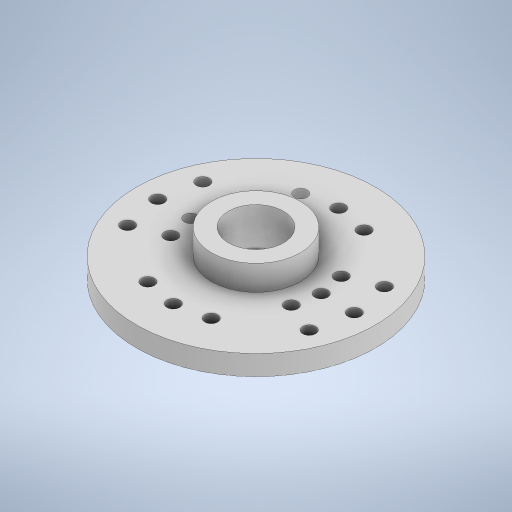
# Autodesk Inventor part: Standard Servo Horn - White Circle
Saved by Autodesk Inventor 2023 (Build 270158000, 158)
## iProperties
Created: 2023-09-05
Part Number: Standard Servo Horn - White Circle
Material: Generic
Document SubType Name: Modeling
Designer: Nate
Density: 1 g/cm^3
Appearance: Default
Author: Nate
Autodesk Inventor part; units mm, degrees
ref_plane "YZ Plane" through (0, 0, 0) normal (1, 0, 0) x (0, 1, 0)
ref_plane "XZ Plane" through (0, 0, 0) normal (0, 1, 0) x (-1, 0, 0)
ref_plane "XY Plane" through (0, 0, 0) normal (0, 0, 1) x (1, 0, 0)
sketch "Sketch1" plane through (0, 0, 0) normal (0, 1, 0) x (-1, 0, 0)
  circle A0 centre (0, 0) radius 11.915
  circle A1 centre (0, 0) radius 9.8
  circle A2 centre (0, 0) radius 8.25
  circle A3 centre (0, 0) radius 6.5
  circle A4 centre (6.5, 0) radius 0.65
  circle A5 centre (9.8, 0) radius 0.65
  circle A6 centre (9.054, 3.7503) radius 0.65
  circle A7 centre (6.0052, 2.4874) radius 0.65
  circle A8 centre (9.054, -3.7503) radius 0.65
  circle A9 centre (6.0052, -2.4874) radius 0.65
  circle A10 centre (-9.054, -3.7503) radius 0.65
  circle A11 centre (-6.0052, -2.4874) radius 0.65
  circle A12 centre (-6.5, 0) radius 0.65
  circle A13 centre (-9.8, 0) radius 0.65
  circle A14 centre (-6.0052, 2.4874) radius 0.65
  circle A15 centre (-9.054, 3.7503) radius 0.65
  circle A16 centre (0, 8.25) radius 0.65
  circle A17 centre (-3.1571, 7.622) radius 0.65
  circle A18 centre (3.1571, 7.622) radius 0.65
  circle A19 centre (-3.1571, -7.622) radius 0.65
  circle A20 centre (0, -8.25) radius 0.65
  circle A21 centre (3.1571, -7.622) radius 0.65
  circle A22 centre (0, 0) radius 1.37
  circle A23 centre (0, 0) radius 2.75
  circle A24 centre (0, 0) radius 2.97
  circle A25 centre (0, 0) radius 3.73
  circle A26 centre (0, 0) radius 4.44
  dimension "d1" = 19.6
  dimension "d2" = 16.5
  dimension "d3" = 13
  dimension "d0" = 23.83
  dimension "d4" = 1.3
  dimension "d5" = 1.3
  dimension "d8" = 22.5
  dimension "d12" = 337.5
  dimension "d16" = 180
  dimension "d18" = 1.3
  dimension "d21" = 22.5
  dimension "d25" = 337.5
  dimension "d29" = 180
  dimension "d31" = 2.74
  dimension "d32" = 5.5
  dimension "d33" = 5.94
  dimension "d34" = 7.46
  dimension "d35" = 8.88
  constraints: 24 centre point, 9 coincident, 2 horizontal alignment, 1 vertical alignment, 42 other
  measures "d0" diameter of A0
  measures "d4" diameter of A4
  measures "d5" diameter of A5
  measures "d18" diameter of A16
  measures "d31" diameter of A22
  measures "d32" diameter of A23
  measures "d33" diameter of A24
  measures "d34" diameter of A25
  measures "d35" diameter of A26
extrude "Extrusion1" add sketch "Sketch1" along normal blind 2 contours A0 | A5 A1 A8 A10 A13 A15 A6 | A2 A21 A20 A19 A17 A16 A18 | A4 A3 A9 A11 A12 A14 A7
extrude "Extrusion2" add sketch "Sketch1" along normal blind 4.5 contours A26
extrude "Extrusion3" add sketch "Sketch1" along normal blind 4.5 and the other way blind 0.5 contours A25
extrude "Extrusion4" add sketch "Sketch1" along normal blind 4.5 contours A24
extrude "Extrusion5" add sketch "Sketch1" along normal blind 0.75 contours A23
body "Solid1"
